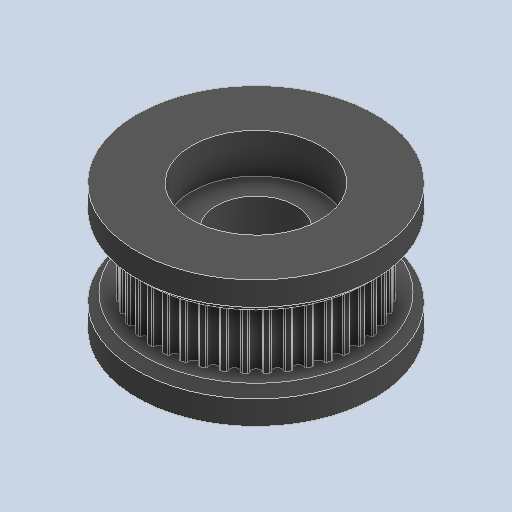
# Autodesk Inventor part: Engranaje Insertado en pin
Saved by Autodesk Inventor 2026 (Build 300175050, 175E)
## iProperties
Created: 2025-07-19
Part Number: Engranaje Insertado en pin
Material: Plastico PETG
Document SubType Name: Modeling
Designer: bello
Density: 1.27 g/cm^3
Appearance: Genérico
Author: bello
Autodesk Inventor part; units mm, degrees
ref_plane "YZ Plane" through (0, 0, 0) normal (1, 0, 0) x (0, 1, 0)
ref_plane "XZ Plane" through (0, 0, 0) normal (0, 1, 0) x (-1, 0, 0)
sketch "Boceto1" plane through (0, 0, 0) normal (0, 1, 0) x (-1, 0, 0)
  circle A0 centre (0, 0) radius 12.4784
  circle A1 centre (0, 0) radius 11.7284
  line L0 (0, 0) -> (0, -12.4784)
  line L1 (0, 0) -> (-1.9521, -12.3248)
  circle A2 centre (0, -12.2834) radius 0.555
  circle A3 centre (-1.9215, -12.1322) radius 0.555
  circle A4 centre (-0.7046, -12.3082) radius 0.15
  circle A5 centre (-1.2295, -12.2669) radius 0.15
  circle A6 centre (0, 0) radius 9.7284
  point P0 (0, -9.7284)
  point P1 (-1.5219, -9.6086)
  point P2 (-1.8347, -11.584)
  point P3 (-1.3768, -12.2383)
  point P4 (-1.2445, -12.4162)
  point P5 (-0.7131, -12.458)
  point P6 (-0.5547, -12.303)
  point P7 (0, -11.7284)
  dimension "d0" = 24.9568
  dimension "d1" = 23.4568
  dimension "d2" = 9
  dimension "d3" = 1.11
  dimension "d4" = 0.3
  dimension "d5" = 19.4568
  constraints: 7 centre point, 6 tangent, 4 end point, 3 coincident, 2 equal radius, 2 point on circle, 2 point on line, 1 vertical
  measures "d0" diameter of A0
  measures "d1" diameter of A1
  measures "d2" angle of L0 L1
  measures "d3" diameter of A2
  measures "d4" diameter of A4
  measures "d5" diameter of A6
extrude "Extrusión1" add sketch "Boceto1" along normal blind 8 contours L1 A6 L0 A1 | A1 A2 A4 A0 A5 A3 | L1 L0 A6 | A5 | A4 picked at (-1.5275, -10.9523) picked at (-0.8463, -6.4279)
pattern_circular "Patrón circular1" count 40 over 360 about axis through (0, -10, 0) along (0, 1, 0) of "Extrusión1"
sketch "Boceto3" plane through (0, 8, 0) normal (0, 1, 0) x (1, 0, 0)
  circle A0 centre (0, 0) radius 15
  dimension "d11" = 30
  constraints: 1 centre point, 1 coincident
  measures "d11" diameter of A0
extrude "Extrusión2" add sketch "Boceto3" along normal blind 4
sketch "Boceto4" plane through (0, 12, 0) normal (0, 1, 0) x (1, 0, 0)
  circle A0 centre (0, 0) radius 5
  dimension "d14" = 10
  constraints: 1 centre point, 1 coincident
  measures "d14" diameter of A0
extrude "Extrusión3" cut sketch "Boceto4" against normal through all
sketch "Boceto5" plane through (0, 12, 0) normal (0, 1, 0) x (1, 0, 0)
  circle A0 centre (0, 0) radius 8.1
  dimension "d17" = 16.2
  constraints: 1 centre point, 1 coincident
  measures "d17" diameter of A0
extrude "Extrusión4" cut sketch "Boceto5" against normal blind 5
ref_plane "Plano de trabajo1" through (0, 4, 0) normal (0, -1, 0) x (1, 0, 0)
mirror "Simetría1" about plane through (0, 4, 0) normal (0, -1, 0) of "Extrusión2", "Extrusión4"
chamfer "Chaflán1" distance 1 angle 45 2 edges at (-15, 8, 0) (-15, 0, 0)
equation "\"d0\" = PitchDiameter"
equation "\"d1\" = InnerDiameter"
equation "\"d2\" = ToothAngle"
equation "\"d3\" = RootDiameter"
equation "\"d4\" = ShoulderDiameter"
equation "\"Pitch\" = 2"
equation "\"InnerDiameter\" = PitchDiameter - 2 * ToothHeight"
equation "\"PitchDiameter\" = PulleyDiameter - 2 * PLD"
equation "\"PLD\" = 0.254"
equation "\"ToothHeight\" = 0.75"
equation "\"ShoulderDiameter\" = 0.3"
equation "\"RootDiameter\" = 1.11"
equation "\"ToothAngle\" = 9deg"
equation "\"PulleyDiameter\" = 25.464791"
